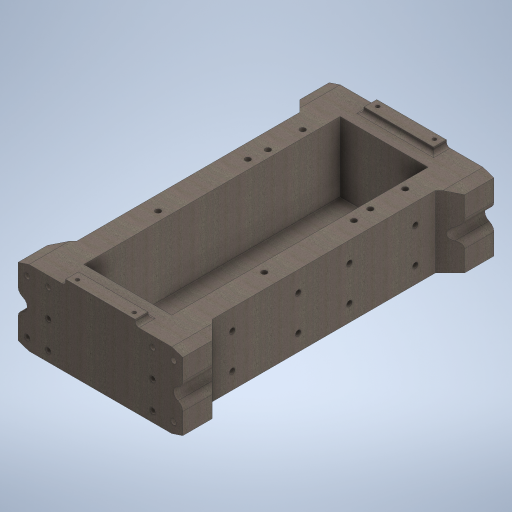
# Autodesk Inventor part: Part1
Saved by Autodesk Inventor 2023 (Build 270158000, 158)
## iProperties
Created: 2023-08-12
Part Number: Part1
Material: ABS Plastic
Document SubType Name: Modeling
Designer: Dawid
Density: 1.06 g/cm^3
Appearance: Walnut
Author: Dawid
Autodesk Inventor part; units mm, degrees
ref_plane "YZ Plane" through (0, 0, 0) normal (1, 0, 0) x (0, 1, 0)
ref_plane "XZ Plane" through (0, 0, 0) normal (0, 1, 0) x (-1, 0, 0)
ref_plane "XY Plane" through (0, 0, 0) normal (0, 0, 1) x (1, 0, 0)
sketch "Sketch1" plane through (0, 0, 0) normal (0, 1, 0) x (-1, 0, 0)
  line L0 (45, 85) -> (-45, 85)
  line L1 (-45, 85) -> (-45, -85)
  line L2 (-45, -85) -> (45, -85)
  line L3 (45, -85) -> (45, 85)
  line L4 (45, 85) -> (-45, -85) construction
  line L5 (-45, 85) -> (45, -85) construction
  line L6 (24, 70) -> (-24, 70)
  line L7 (-24, 70) -> (-24, -70)
  line L8 (-24, -70) -> (24, -70)
  line L9 (24, -70) -> (24, 70)
  line L10 (24, 70) -> (-24, -70) construction
  line L11 (-24, 70) -> (24, -70) construction
  point P0 (0, 0)
  dimension "d0" = 90
  dimension "d1" = 170
  dimension "d2" = 48
  dimension "d3" = 140
  constraints: 24 end point, 4 midpoint, 4 parallel, 2 horizontal, 2 perpendicular
  measures "d0" distance of L2.end L1.end
  measures "d1" distance of L1.end L0.end
  measures "d2" distance of L8.end L7.end
  measures "d3" distance of L7.end L6.end
extrude "Extrusion1" add sketch "Sketch1" along normal blind 38
sketch "Sketch2" plane through (0, 0, 0) normal (0, -1, 0) x (1, 0, 0)
  line L0 (45, 85) -> (45, -85) projected
  line L1 (-45, -85) -> (-45, 85) projected
  line L2 (45, 85) -> (-45, 85)
  line L3 (-45, 85) -> (-45, -85)
  line L4 (-45, -85) -> (45, -85)
  line L5 (45, -85) -> (45, 85)
  point P0 (0, 0)
  constraints: 8 end point, 2 parallel, 1 horizontal, 1 perpendicular
extrude "Extrusion2" add sketch "Sketch2" along normal blind 3
sketch "Sketch4" plane through (0, 38, 0) normal (0, 1, 0) x (1, 0, 0)
  line L0 (-29, -24.5) -> (29, -24.5)
  line L1 (29, -24.5) -> (29, 24.5)
  line L2 (29, 24.5) -> (-29, 24.5)
  line L3 (-29, 24.5) -> (-29, -24.5)
  line L4 (-29, -24.5) -> (29, 24.5) construction
  line L5 (29, -24.5) -> (-29, 24.5) construction
  circle A0 centre (-29, -24.5) radius 1.5
  circle A1 centre (-29, 24.5) radius 1.5
  circle A2 centre (29, 24.5) radius 1.5
  circle A3 centre (29, -24.5) radius 1.5
  point P0 (0, 0)
  dimension "d8" = 58
  dimension "d9" = 49
  dimension "d10" = 3
  dimension "d11" = 3
  dimension "d12" = 3
  dimension "d13" = 3
  constraints: 12 end point, 4 centre point, 4 coincident, 2 midpoint, 2 parallel, 1 horizontal, 1 perpendicular
  measures "d8" distance of L2.end L1.end
  measures "d9" distance of L1.end L0.end
  measures "d10" diameter of A0
  measures "d11" diameter of A1
  measures "d12" diameter of A2
  measures "d13" diameter of A3
extrude "Extrusion3" cut sketch "Sketch4" against normal blind 7 contours L3 A0 L0 | L0 A0 L3 | A3 L1 L0 | L0 L1 A3 | A1 L2 L3 | L3 L2 A1 | A2 L2 L1 | L1 L2 A2
sketch "Sketch5" plane through (0, 38, 0) normal (0, 1, 0) x (1, 0, 0)
  line L0 (0, 0) -> (0, 24.5)
  line L1 (0, 24.5) -> (0, 34.5)
  line L2 (0, 34.5) -> (-28, 34.5)
  line L3 (-28, 34.5) -> (28, 34.5)
  line L4 (28, 34.5) -> (28, 53.5)
  line L5 (28, 53.5) -> (-28, 53.5)
  line L6 (-28, 53.5) -> (-28, 34.5)
  circle A0 centre (-28, 34.5) radius 1.5
  circle A1 centre (-28, 53.5) radius 1.5
  circle A2 centre (28, 53.5) radius 1.5
  circle A3 centre (28, 34.5) radius 1.5
  dimension "d16" = 10
  dimension "d17" = 28
  dimension "d18" = 56
  dimension "d19" = 19
  dimension "d20" = 3
  dimension "d21" = 3
  dimension "d22" = 3
  dimension "d23" = 3
  constraints: 14 end point, 4 centre point, 4 coincident, 4 perpendicular, 2 point on line, 1 vertical
  measures "d16" distance of L0.end L1.end
  measures "d17" distance of L1.end L2.end
  measures "d18" distance of L2.end L3.end
  measures "d19" distance of L3.end L4.end
  measures "d20" diameter of A0
  measures "d21" diameter of A1
  measures "d22" diameter of A2
  measures "d23" diameter of A3
extrude "Extrusion4" cut sketch "Sketch5" against normal blind 7 contours A0 L6 L2 | L2 L6 A0 | A3 L4 L3 | L3 L4 A3 | A1 L5 L6 | L6 L5 A1 | A2 L5 L4 | L4 L5 A2
sketch "Sketch7" plane through (45, 38, -85) normal (0, 0, -1) x (-1, 0, 0)
  line L0 (90, -41) -> (90, 0) projected
  line L1 (90, -41) -> (0, -41) projected
  line L2 (21.5, 0) -> (68.5, 0)
  line L3 (68.5, 0) -> (68.5, -41)
  line L4 (68.5, -41) -> (21.5, -41)
  line L5 (21.5, -41) -> (21.5, 0)
  line L6 (21.5, 0) -> (68.5, -41) construction
  line L7 (68.5, 0) -> (21.5, -41) construction
  line L8 (0, 0) -> (90, 0)
  line L9 (90, 0) -> (90, -41)
  line L10 (90, -41) -> (0, -41)
  line L11 (0, -41) -> (0, 0)
  line L12 (0, 0) -> (90, -41) construction
  line L13 (90, 0) -> (0, -41) construction
  line L14 (11.5, 0) -> (78.5, 0)
  line L15 (78.5, 0) -> (78.5, -41)
  line L16 (78.5, -41) -> (11.5, -41)
  line L17 (11.5, -41) -> (11.5, 0)
  line L18 (11.5, 0) -> (78.5, -41) construction
  line L19 (78.5, 0) -> (11.5, -41) construction
  line L20 (0, 0) -> (0, -20.5)
  line L21 (0, -41) -> (0, 0) projected
  line L22 (0, -20.5) -> (90, -20.5)
  line L23 (-8.5, 0) -> (98.5, 0)
  line L24 (98.5, 0) -> (98.5, -41)
  line L25 (98.5, -41) -> (-8.5, -41)
  line L26 (-8.5, -41) -> (-8.5, 0)
  line L27 (-8.5, 0) -> (98.5, -41) construction
  line L28 (98.5, 0) -> (-8.5, -41) construction
  line L29 (-8.5, 0) -> (1.5, 0)
  line L30 (0, 0) -> (90, 0) projected
  line L31 (1.5, 0) -> (1.5, -41)
  line L32 (98.5, -41) -> (88.5, -41)
  line L33 (88.5, -41) -> (88.5, 0)
  circle A0 centre (1.5, -20.5) radius 10
  circle A1 centre (88.5, -20.5) radius 10
  line L34 (21.5, -41) -> (16.5, -41)
  line L35 (16.5, -41) -> (16.5, 0)
  line L36 (16.5, -20.5) -> (16.5, -35.5)
  line L37 (16.5, -35.5) -> (16.5, -5.5)
  circle A2 centre (16.5, -5.5) radius 1.5
  circle A3 centre (16.5, -35.5) radius 1.5
  circle A4 centre (16.5, -20.5) radius 1.5
  line L38 (0, 0) -> (5, 0)
  line L39 (5, 0) -> (5, -6)
  line L40 (0, -41) -> (5, -41)
  line L41 (5, -41) -> (5, -35)
  circle A5 centre (5, -35) radius 1.5
  circle A6 centre (5, -6) radius 1.5
  line L42 (68.5, -20.5) -> (73.5, -20.5)
  line L43 (73.5, -20.5) -> (73.5, -35.5)
  line L44 (73.5, -35.5) -> (73.5, -5.5)
  line L45 (90, 0) -> (85, 0)
  line L46 (85, 0) -> (85, -6)
  line L47 (90, -41) -> (85, -41)
  line L48 (85, -41) -> (85, -35)
  circle A7 centre (73.5, -5.5) radius 1.5
  circle A8 centre (73.5, -20.5) radius 1.5
  circle A9 centre (73.5, -35.5) radius 1.5
  circle A10 centre (85, -35) radius 1.5
  circle A11 centre (85, -6) radius 1.5
  point P0 (45, -38)
  point P1 (45, -20.5)
  point P2 (45, -20.5)
  dimension "d27" = 47
  dimension "d28" = 67
  dimension "d29" = 107
  dimension "d30" = 10
  dimension "d31" = 10
  dimension "d32" = 5
  dimension "d33" = 15
  dimension "d34" = 30
  dimension "d35" = 3
  dimension "d36" = 3
  dimension "d37" = 3
  dimension "d38" = 5
  dimension "d39" = 6
  dimension "d40" = 5
  dimension "d41" = 6
  dimension "d42" = 3
  dimension "d43" = 3
  dimension "d44" = 5
  dimension "d45" = 15
  dimension "d46" = 30
  dimension "d47" = 5
  dimension "d48" = 6
  dimension "d49" = 5
  dimension "d50" = 6
  dimension "d51" = 3
  dimension "d52" = 3
  dimension "d53" = 3
  dimension "d54" = 3
  dimension "d55" = 3
  constraints: 90 end point, 14 midpoint, 13 point on line, 12 centre point, 11 perpendicular, 10 coincident, 8 parallel, 4 horizontal, 1 tangent, 1 vertical, 5 other
  measures "d27" distance of L3.end L4.end
  measures "d28" distance of L15.end L16.end
  measures "d29" distance of L24.end L25.end
  measures "d30" distance of L23.start L29.end
  measures "d31" distance of L24.end L32.end
  measures "d32" distance of L4.end L34.end
  measures "d33" distance of L36.start L36.end
  measures "d34" distance of L36.end L37.end
  measures "d35" diameter of A2
  measures "d36" diameter of A3
  measures "d37" diameter of A4
  measures "d38" distance of L20.start L38.end
  measures "d39" distance of L38.end L39.end
  measures "d40" distance of L10.end L40.end
  measures "d41" distance of L40.end L41.end
  measures "d42" diameter of A5
  measures "d43" diameter of A6
  measures "d44" distance of L42.start L42.end
  measures "d45" distance of L42.end L43.end
  measures "d46" distance of L43.end L44.end
  measures "d47" distance of L8.end L45.end
  measures "d48" distance of L45.end L46.end
  measures "d49" distance of L0.start L47.end
  measures "d50" distance of L47.end L48.end
  measures "d51" diameter of A7
  measures "d52" diameter of A8
  measures "d53" diameter of A9
  measures "d54" diameter of A10
  measures "d55" diameter of A11
extrude "Extrusion5" cut sketch "Sketch7" against normal blind 8 contours A8 L43 L22 | L22 L44 A8 | L43 A8 L22 | L22 A8 L44 | A3 L35 | L35 A3 | A4 L35 L22 | L22 L35 A4 | A2 L35 | L35 A2 | L35 A4 L22 | L22 A4 L35 | A5 | A6 | A7 | A9 | A10 | A11
sketch "Sketch8" plane through (-45, 38, 85) normal (0, 0, 1) x (1, 0, 0)
  line L0 (90, -41) -> (90, 0)
  line L1 (90, -41) -> (0, -41)
  line L2 (21.5, 0) -> (68.5, 0)
  line L3 (68.5, 0) -> (68.5, -41)
  line L4 (68.5, -41) -> (21.5, -41)
  line L5 (21.5, -41) -> (21.5, 0)
  line L6 (21.5, 0) -> (68.5, -41) construction
  line L7 (68.5, 0) -> (21.5, -41) construction
  line L8 (0, 0) -> (90, 0)
  line L9 (90, 0) -> (90, -41)
  line L10 (90, -41) -> (0, -41)
  line L11 (0, -41) -> (0, 0)
  line L12 (0, 0) -> (90, -41) construction
  line L13 (90, 0) -> (0, -41) construction
  line L14 (11.5, 0) -> (78.5, 0)
  line L15 (78.5, 0) -> (78.5, -41)
  line L16 (78.5, -41) -> (11.5, -41)
  line L17 (11.5, -41) -> (11.5, 0)
  line L18 (11.5, 0) -> (78.5, -41) construction
  line L19 (78.5, 0) -> (11.5, -41) construction
  line L20 (0, 0) -> (0, -20.5)
  line L21 (0, -41) -> (0, 0)
  line L22 (0, -20.5) -> (90, -20.5)
  line L23 (-8.5, 0) -> (98.5, 0)
  line L24 (98.5, 0) -> (98.5, -41)
  line L25 (98.5, -41) -> (-8.5, -41)
  line L26 (-8.5, -41) -> (-8.5, 0)
  line L27 (-8.5, 0) -> (98.5, -41) construction
  line L28 (98.5, 0) -> (-8.5, -41) construction
  line L29 (-8.5, 0) -> (1.5, 0)
  line L30 (0, 0) -> (90, 0)
  line L31 (1.5, 0) -> (1.5, -41)
  line L32 (98.5, -41) -> (88.5, -41)
  line L33 (88.5, -41) -> (88.5, 0)
  circle A0 centre (1.5, -20.5) radius 10
  circle A1 centre (88.5, -20.5) radius 10
  line L34 (21.5, -41) -> (16.5, -41)
  line L35 (16.5, -41) -> (16.5, 0)
  line L36 (16.5, -20.5) -> (16.5, -35.5)
  line L37 (16.5, -35.5) -> (16.5, -5.5)
  circle A2 centre (16.5, -5.5) radius 1.5
  circle A3 centre (16.5, -35.5) radius 1.5
  circle A4 centre (16.5, -20.5) radius 1.5
  line L38 (0, 0) -> (5, 0)
  line L39 (5, 0) -> (5, -6)
  line L40 (0, -41) -> (5, -41)
  line L41 (5, -41) -> (5, -35)
  circle A5 centre (5, -35) radius 1.5
  circle A6 centre (5, -6) radius 1.5
  line L42 (68.5, -20.5) -> (73.5, -20.5)
  line L43 (73.5, -20.5) -> (73.5, -35.5)
  line L44 (73.5, -35.5) -> (73.5, -5.5)
  line L45 (90, 0) -> (85, 0)
  line L46 (85, 0) -> (85, -6)
  line L47 (90, -41) -> (85, -41)
  line L48 (85, -41) -> (85, -35)
  circle A7 centre (73.5, -5.5) radius 1.5
  circle A8 centre (73.5, -20.5) radius 1.5
  circle A9 centre (73.5, -35.5) radius 1.5
  circle A10 centre (85, -35) radius 1.5
  circle A11 centre (85, -6) radius 1.5
  point P0 (45, -38)
  point P1 (45, -38)
  point P2 (45, -20.5)
  point P3 (45, -20.5)
  dimension "d58" = 47
  dimension "d59" = 67
  dimension "d60" = 107
  dimension "d61" = 10
  dimension "d62" = 10
  dimension "d63" = 5
  dimension "d64" = 15
  dimension "d65" = 30
  dimension "d66" = 3
  dimension "d67" = 3
  dimension "d68" = 3
  dimension "d69" = 5
  dimension "d70" = 6
  dimension "d71" = 5
  dimension "d72" = 6
  dimension "d73" = 3
  dimension "d74" = 3
  dimension "d75" = 5
  dimension "d76" = 15
  dimension "d77" = 30
  dimension "d78" = 5
  dimension "d79" = 6
  dimension "d80" = 5
  dimension "d81" = 6
  dimension "d82" = 3
  dimension "d83" = 3
  dimension "d84" = 3
  dimension "d85" = 3
  dimension "d86" = 3
  constraints: 96 end point, 14 midpoint, 13 point on line, 12 centre point, 11 perpendicular, 10 coincident, 8 parallel, 4 horizontal, 1 tangent, 1 vertical, 7 other
  measures "d58" distance of L6.end L7.end
  measures "d59" distance of L15.end L19.end
  measures "d60" distance of L24.end L28.end
  measures "d61" distance of L27.start L31.start
  measures "d62" distance of L24.end L33.start
  measures "d63" distance of L7.end L35.start
  measures "d64" distance of L36.start L37.start
  measures "d65" distance of L37.start L37.end
  measures "d66" diameter of A2
  measures "d67" diameter of A3
  measures "d68" diameter of A4
  measures "d69" distance of L20.start L39.start
  measures "d70" distance of L39.start L39.end
  measures "d71" distance of L10.end L40.end
  measures "d72" distance of L40.end L41.end
  measures "d73" diameter of A5
  measures "d74" diameter of A6
  measures "d75" distance of L42.start L42.end
  measures "d76" distance of L42.end L44.start
  measures "d77" distance of L44.start L44.end
  measures "d78" distance of L9.start L46.start
  measures "d79" distance of L46.start L46.end
  measures "d80" distance of L0.start L48.start
  measures "d81" distance of L48.start L48.end
  measures "d82" diameter of A7
  measures "d83" diameter of A8
  measures "d84" diameter of A9
  measures "d85" diameter of A10
  measures "d86" diameter of A11
extrude "Extrusion6" cut sketch "Sketch8" against normal blind 8 contours A8 L43 L22 | L22 L44 A8 | L43 A8 L22 | L22 A8 L44 | A3 L35 | L35 A3 | A4 L35 L22 | L22 L35 A4 | A2 L35 | L35 A2 | L35 A4 L22 | L22 A4 L35 | A5 | A6 | A7 | A9 | A10 | A11
sketch "Sketch10" plane through (-45, 38, -85) normal (-1, 0, 0) x (0, 0, 1)
  line L0 (0, -41) -> (0, 0) projected
  line L1 (0, 0) -> (85, 0)
  line L2 (15, 0) -> (155, 0) projected
  line L3 (0, -41) -> (170, -41) projected
  line L4 (15, -38) -> (15, 0) projected
  line L5 (25, 0) -> (145, 0)
  line L6 (145, -41) -> (25, -41)
  line L7 (20, 0) -> (150, 0)
  line L8 (150, 0) -> (150, -41)
  line L9 (150, -41) -> (20, -41)
  line L10 (20, -41) -> (20, 0)
  point P0 (85, -38)
  dimension "d91" = 130
  constraints: 14 end point, 3 parallel, 2 horizontal, 2 point on line, 1 midpoint, 1 perpendicular
  measures "d91" distance of L8.end L9.end
extrude "Extrusion7" cut sketch "Sketch10" against normal blind 8 contours L10 L1 L2 L8 L3
chamfer "Chamfer1" distance 4 angle 45 4 edges at (-37, 17.5, -65) (-37, 17.5, 65) (-45, 17.5, 65) (-45, 17.5, -65)
sketch "Sketch11" plane through (45, 38, 85) normal (1, 0, 0) x (0, 0, -1)
  line L0 (170, -41) -> (0, -41) projected
  line L1 (170, -41) -> (170, 0) projected
  line L2 (170, -41) -> (170, 0)
  line L3 (170, 0) -> (170, -20.5)
  line L4 (170, -20.5) -> (0, -20.5)
  line L5 (0, -41) -> (0, 0) projected
  line L6 (0, 0) -> (170, 0) projected
  line L7 (150, -41) -> (20, -41)
  line L8 (20, -41) -> (20, 0)
  line L9 (20, 0) -> (150, 0)
  line L10 (150, 0) -> (150, -41)
  line L11 (150, -41) -> (20, 0) construction
  line L12 (20, -41) -> (150, 0) construction
  point P0 (85, -38)
  point P1 (85, -20.5)
  dimension "d97" = 130
  constraints: 18 end point, 5 midpoint, 3 equal length, 1 horizontal, 1 perpendicular, 1 point on line
  measures "d97" distance of L8.end L9.end
extrude "Extrusion8" cut sketch "Sketch11" against normal blind 8 contours L0 L8 L4 L10 | L4 L8 L6 L10
chamfer "Chamfer2" distance 4 angle 45 4 edges at (37, 17.5, -65) (45, 17.5, -65) (45, 17.5, 65) (37, 17.5, 65)
sketch "Sketch13" plane through (37, 38, 85) normal (1, 0, 0) x (0, 0, -1)
  line L0 (0, 0) -> (16, 0) projected
  line L1 (0, 0) -> (0, -20.5)
  line L2 (0, -41) -> (0, 0) projected
  line L3 (0, -20.5) -> (170, -20.5)
  line L4 (85, -20.5) -> (85, -41)
  line L5 (24, -41) -> (146, -41) projected
  line L6 (85, -20.5) -> (90, -20.5)
  line L7 (90, -20.5) -> (80, -20.5)
  line L8 (26, -8.5) -> (144, -8.5)
  line L9 (144, -8.5) -> (144, -32.5)
  line L10 (144, -32.5) -> (26, -32.5)
  line L11 (26, -32.5) -> (26, -8.5)
  line L12 (26, -8.5) -> (144, -32.5) construction
  line L13 (144, -8.5) -> (26, -32.5) construction
  line L14 (80, -8.5) -> (90, -8.5)
  line L15 (90, -8.5) -> (90, -32.5)
  line L16 (90, -32.5) -> (80, -32.5)
  line L17 (80, -32.5) -> (80, -8.5)
  line L18 (80, -8.5) -> (90, -32.5) construction
  line L19 (90, -8.5) -> (80, -32.5) construction
  line L20 (80, -32.5) -> (80, -30)
  line L21 (80, -30) -> (71, -30)
  line L22 (80, -8.5) -> (80, -11)
  line L23 (80, -11) -> (71, -11)
  line L24 (26, -8.5) -> (26, -11)
  line L25 (26, -11) -> (35, -11)
  line L26 (26, -32.5) -> (26, -30)
  line L27 (26, -30) -> (35, -30)
  line L28 (90, -8.5) -> (90, -11)
  line L29 (90, -11) -> (99, -11)
  line L30 (90, -32.5) -> (90, -30)
  line L31 (90, -30) -> (99, -30)
  line L32 (144, -32.5) -> (144, -30)
  line L33 (144, -30) -> (135, -30)
  line L34 (144, -8.5) -> (144, -11)
  line L35 (144, -11) -> (135, -11)
  circle A0 centre (35, -11) radius 1.5
  circle A1 centre (35, -30) radius 1.5
  circle A2 centre (71, -30) radius 1.5
  circle A3 centre (71, -11) radius 1.5
  circle A4 centre (99, -11) radius 1.5
  circle A5 centre (135, -11) radius 1.5
  circle A6 centre (99, -30) radius 1.5
  circle A7 centre (135, -30) radius 1.5
  point P0 (85, -38)
  dimension "d103" = 5
  dimension "d104" = 10
  dimension "d105" = 118
  dimension "d106" = 24
  dimension "d107" = 2.5
  dimension "d108" = 9
  dimension "d109" = 2.5
  dimension "d110" = 9
  dimension "d111" = 2.5
  dimension "d112" = 9
  dimension "d113" = 2.5
  dimension "d114" = 9
  dimension "d115" = 2.5
  dimension "d116" = 9
  dimension "d117" = 2.5
  dimension "d118" = 9
  dimension "d119" = 2.5
  dimension "d120" = 9
  dimension "d121" = 2.5
  dimension "d122" = 9
  dimension "d123" = 3
  dimension "d124" = 3
  dimension "d125" = 3
  dimension "d126" = 3
  dimension "d127" = 3
  dimension "d128" = 3
  dimension "d129" = 3
  dimension "d130" = 3
  constraints: 66 end point, 11 point on line, 9 perpendicular, 8 centre point, 8 coincident, 7 midpoint, 5 parallel, 3 horizontal
  measures "d103" distance of L4.start L6.end
  measures "d104" distance of L6.end L7.end
  measures "d105" distance of L9.end L10.end
  measures "d106" distance of L8.end L9.end
  measures "d107" distance of L16.end L20.end
  measures "d108" distance of L20.end L21.end
  measures "d109" distance of L14.start L22.end
  measures "d110" distance of L22.end L23.end
  measures "d111" distance of L8.start L24.end
  measures "d112" distance of L24.end L25.end
  measures "d113" distance of L10.end L26.end
  measures "d114" distance of L26.end L27.end
  measures "d115" distance of L14.end L28.end
  measures "d116" distance of L28.end L29.end
  measures "d117" distance of L15.end L30.end
  measures "d118" distance of L30.end L31.end
  measures "d119" distance of L9.end L32.end
  measures "d120" distance of L32.end L33.end
  measures "d121" distance of L8.end L34.end
  measures "d122" distance of L34.end L35.end
  measures "d123" diameter of A0
  measures "d124" diameter of A1
  measures "d125" diameter of A2
  measures "d126" diameter of A3
  measures "d127" diameter of A4
  measures "d128" diameter of A5
  measures "d129" diameter of A6
  measures "d130" diameter of A7
extrude "Extrusion9" cut sketch "Sketch13" against normal blind 5 contours A0 | A1 | A2 | A3 | A4 | A5 | A6 | A7
sketch "Sketch14" plane through (-37, 38, -85) normal (-1, 0, 0) x (0, 0, 1)
  line L0 (0, 0) -> (16, 0)
  line L1 (0, 0) -> (0, -20.5)
  line L2 (0, -41) -> (0, 0)
  line L3 (0, -20.5) -> (170, -20.5)
  line L4 (85, -20.5) -> (85, -41)
  line L5 (24, -41) -> (146, -41)
  line L6 (85, -20.5) -> (90, -20.5)
  line L7 (90, -20.5) -> (80, -20.5)
  line L8 (26, -8.5) -> (144, -8.5)
  line L9 (144, -8.5) -> (144, -32.5)
  line L10 (144, -32.5) -> (26, -32.5)
  line L11 (26, -32.5) -> (26, -8.5)
  line L12 (26, -8.5) -> (144, -32.5) construction
  line L13 (144, -8.5) -> (26, -32.5) construction
  line L14 (80, -8.5) -> (90, -8.5)
  line L15 (90, -8.5) -> (90, -32.5)
  line L16 (90, -32.5) -> (80, -32.5)
  line L17 (80, -32.5) -> (80, -8.5)
  line L18 (80, -8.5) -> (90, -32.5) construction
  line L19 (90, -8.5) -> (80, -32.5) construction
  line L20 (80, -32.5) -> (80, -30)
  line L21 (80, -30) -> (71, -30)
  line L22 (80, -8.5) -> (80, -11)
  line L23 (80, -11) -> (71, -11)
  line L24 (26, -8.5) -> (26, -11)
  line L25 (26, -11) -> (35, -11)
  line L26 (26, -32.5) -> (26, -30)
  line L27 (26, -30) -> (35, -30)
  line L28 (90, -8.5) -> (90, -11)
  line L29 (90, -11) -> (99, -11)
  line L30 (90, -32.5) -> (90, -30)
  line L31 (90, -30) -> (99, -30)
  line L32 (144, -32.5) -> (144, -30)
  line L33 (144, -30) -> (135, -30)
  line L34 (144, -8.5) -> (144, -11)
  line L35 (144, -11) -> (135, -11)
  circle A0 centre (35, -11) radius 1.5
  circle A1 centre (35, -30) radius 1.5
  circle A2 centre (71, -30) radius 1.5
  circle A3 centre (71, -11) radius 1.5
  circle A4 centre (99, -11) radius 1.5
  circle A5 centre (135, -11) radius 1.5
  circle A6 centre (99, -30) radius 1.5
  circle A7 centre (135, -30) radius 1.5
  point P0 (85, -38)
  point P1 (85, -38)
  dimension "d133" = 5
  dimension "d134" = 10
  dimension "d135" = 118
  dimension "d136" = 24
  dimension "d137" = 2.5
  dimension "d138" = 9
  dimension "d139" = 2.5
  dimension "d140" = 9
  dimension "d141" = 2.5
  dimension "d142" = 9
  dimension "d143" = 2.5
  dimension "d144" = 9
  dimension "d145" = 2.5
  dimension "d146" = 9
  dimension "d147" = 2.5
  dimension "d148" = 9
  dimension "d149" = 2.5
  dimension "d150" = 9
  dimension "d151" = 2.5
  dimension "d152" = 9
  dimension "d153" = 3
  dimension "d154" = 3
  dimension "d155" = 3
  dimension "d156" = 3
  dimension "d157" = 3
  dimension "d158" = 3
  dimension "d159" = 3
  dimension "d160" = 3
  constraints: 72 end point, 11 point on line, 9 perpendicular, 8 centre point, 8 coincident, 7 midpoint, 5 parallel, 3 horizontal
  measures "d133" distance of L4.start L7.start
  measures "d134" distance of L7.start L7.end
  measures "d135" distance of L12.end L10.end
  measures "d136" distance of L8.end L12.end
  measures "d137" distance of L17.start L20.end
  measures "d138" distance of L20.end L21.end
  measures "d139" distance of L14.start L22.end
  measures "d140" distance of L22.end L23.end
  measures "d141" distance of L8.start L25.start
  measures "d142" distance of L25.start L25.end
  measures "d143" distance of L10.end L26.end
  measures "d144" distance of L26.end L27.end
  measures "d145" distance of L14.end L28.end
  measures "d146" distance of L28.end L29.end
  measures "d147" distance of L18.end L31.start
  measures "d148" distance of L31.start L31.end
  measures "d149" distance of L12.end L32.end
  measures "d150" distance of L32.end L33.end
  measures "d151" distance of L8.end L34.end
  measures "d152" distance of L34.end L35.end
  measures "d153" diameter of A0
  measures "d154" diameter of A1
  measures "d155" diameter of A2
  measures "d156" diameter of A3
  measures "d157" diameter of A4
  measures "d158" diameter of A5
  measures "d159" diameter of A6
  measures "d160" diameter of A7
extrude "Extrusion10" cut sketch "Sketch14" against normal blind 5 contours A0 | A1 | A2 | A3 | A4 | A5 | A6 | A7
sketch "Sketch15" plane through (0, 38, 0) normal (0, 1, 0) x (1, 0, 0)
  line L0 (45, -85) -> (-45, -85) projected
  line L1 (-45, -85) -> (45, -85)
  line L2 (0, -85) -> (0, -78)
  line L3 (0, -78) -> (-19, -78)
  line L4 (-19, -78) -> (19, -78)
  line L5 (19, -78) -> (19, -85)
  line L6 (-19, -78) -> (-19, -85)
  point P0 (0, 0)
  dimension "d163" = 7
  dimension "d164" = 19
  dimension "d165" = 38
  constraints: 12 end point, 3 perpendicular, 3 point on line, 1 collinear, 1 midpoint, 1 vertical
  measures "d163" distance of L2.start L2.end
  measures "d164" distance of L2.end L3.end
  measures "d165" distance of L3.end L4.end
extrude "Extrusion11" add sketch "Sketch15" along normal blind 3
sketch "Sketch16" plane through (0, 38, 0) normal (0, 1, 0) x (1, 0, 0)
  line L0 (45, -85) -> (-45, -85)
  line L1 (-45, -85) -> (45, -85)
  line L2 (0, -85) -> (0, -78)
  line L3 (0, -78) -> (-19, -78)
  line L4 (-19, -78) -> (19, -78)
  line L5 (19, -78) -> (19, -85)
  line L6 (-19, -78) -> (-19, -85)
  line L7 (45, 85) -> (-45, 85) projected
  line L8 (0, 85) -> (0, 78)
  line L9 (0, 78) -> (19, 78)
  line L10 (19, 78) -> (-19, 78)
  line L11 (-19, 78) -> (-19, 85)
  line L12 (19, 78) -> (19, 85)
  point P0 (0, 0)
  dimension "d168" = 7
  dimension "d169" = 19
  dimension "d170" = 38
  dimension "d171" = 7
  dimension "d172" = 19
  dimension "d173" = 38
  constraints: 24 end point, 6 point on line, 5 perpendicular, 2 equal length, 2 midpoint, 2 vertical
  measures "d168" distance of L2.start L2.end
  measures "d169" distance of L2.end L3.end
  measures "d170" distance of L3.end L4.end
  measures "d171" distance of L8.start L8.end
  measures "d172" distance of L8.end L9.end
  measures "d173" distance of L9.end L10.end
extrude "Extrusion12" add sketch "Sketch16" along normal blind 3 contours L12 L9 L8 L7 | L8 L10 L11 L7
sketch "Sketch17" plane through (0, 41, 0) normal (0, 1, 0) x (1, 0, 0)
  line L0 (45, -85) -> (-45, -85) projected
  line L1 (0, -85) -> (0, -82)
  line L2 (0, -82) -> (-15.5, -82)
  line L3 (-15.5, -82) -> (15.5, -82)
  circle A0 centre (-15.5, -82) radius 1
  circle A1 centre (15.5, -82) radius 1
  line L4 (-45, 85) -> (45, 85) projected
  line L5 (0, 85) -> (0, 82)
  line L6 (0, 82) -> (-15.5, 82)
  line L7 (-15.5, 82) -> (15.5, 82)
  circle A2 centre (-15.5, 82) radius 1
  circle A3 centre (15.5, 82) radius 1
  point P0 (0, 0)
  dimension "d176" = 3
  dimension "d177" = 15.5
  dimension "d178" = 31
  dimension "d179" = 2
  dimension "d180" = 2
  dimension "d181" = 3
  dimension "d182" = 15.5
  dimension "d183" = 31
  dimension "d184" = 2
  dimension "d185" = 2
  constraints: 12 end point, 4 centre point, 4 coincident, 2 midpoint, 2 perpendicular, 2 point on line, 2 vertical
  measures "d176" distance of L1.start L1.end
  measures "d177" distance of L1.end L2.end
  measures "d178" distance of L2.end L3.end
  measures "d179" diameter of A0
  measures "d180" diameter of A1
  measures "d181" distance of L5.start L5.end
  measures "d182" distance of L5.end L6.end
  measures "d183" distance of L6.end L7.end
  measures "d184" diameter of A2
  measures "d185" diameter of A3
extrude "Extrusion13" cut sketch "Sketch17" against normal blind 6
chamfer "Chamfer3" distance 6 distance2 2 18 edges at (37, -3, 0) (43.0001, -3, 66.9999) (41, -3, 65) (39, -3, 63.0001) (39, -3, -63.0001) (41, -3, -65) (43.0001, -3, -66.9999) (45, -3, -76.9999) (45, -3, 77) (-37, -3, 0) (-39, -3, -63.0001) (-41, -3, -65) (-43.0001, -3, -66.9999) (-45, -3, -77) (-45, -3, 76.9999) (-43.0001, -3, 66.9999) (-41, -3, 65) (-39, -3, 63.0001) measured on face at (38.6464, -3, 63.3536) measured on face at (-38.6464, -3, 63.3536) measured on face at (-41, -3, -65.5) measured on face at (36.5, -3, 0) measured on face at (-42.6465, -3, -67.3535) measured on face at (42.6465, -3, -67.3535) measured on face at (-36.5, -3, 0) measured on face at (41, -3, -65.5) measured on face at (-44.5, -3, -77) measured on face at (42.6465, -3, 67.3535) measured on face at (-42.6465, -3, 67.3535) measured on face at (-44.5, -3, 77) measured on face at (44.5, -3, -77) measured on face at (-38.6464, -3, -63.3536) measured on face at (44.5, -3, 77) measured on face at (-41, -3, 65.5) measured on face at (38.6464, -3, -63.3536) measured on face at (41, -3, 65.5)
sketch "Sketch20" plane through (-19, 41, 85) normal (0, 0, 1) x (1, 0, 0)
  circle A0 centre (-9.5, -23.5) radius 1.5 projected
  line L0 (-9.5, -23.5) -> (-24.5, -23.5)
  circle A1 centre (-24.5, -23.5) radius 10
  circle A2 centre (47.5, -23.5) radius 1.5 projected
  line L1 (47.5, -23.5) -> (62.5, -23.5)
  circle A3 centre (62.5, -23.5) radius 10
  circle A4 centre (-24.5, -23.5) radius 3.5
  circle A5 centre (62.5, -23.5) radius 3.5
  point P0 (19, -41)
  dimension "d191" = 15
  dimension "d192" = 20
  dimension "d193" = 15
  dimension "d194" = 20
  dimension "d195" = 7
  dimension "d196" = 7
  constraints: 4 centre point, 4 coincident, 4 end point, 2 horizontal
  measures "d191" distance of L0.start L0.end
  measures "d192" diameter of A1
  measures "d193" distance of L1.start L1.end
  measures "d194" diameter of A3
  measures "d195" diameter of A4
  measures "d196" diameter of A5
extrude "Extrusion14" cut sketch "Sketch20" against normal blind 200 contours A4 | A5
fillet "Fillet1" radius 4 8 edges at (45, 20.6623, 76.9999) (45, 14.3377, 76.9999) (45, 14.3377, -77) (45, 20.6623, -77) (-45, 20.6623, 76.9999) (-45, 14.3377, 76.9999) (-45, 20.6623, -77) (-45, 14.3377, -77)
chamfer "Chamfer4" distance 6 distance2 2 4 edges at (45, 38, 76.9999) (45, 38, -77) (-45, 38, -76.9999) (-45, 38, 77) measured on face at (44.5, 38, 77) measured on face at (-44.5, 38, 77) measured on face at (-44.5, 38, -77) measured on face at (44.5, 38, -77)
fillet "Fillet2" radius 2 3 edges at (-19, 38, 81.5) (0, 38, 78) (19, 38, 81.5)
fillet "Fillet3" radius 2 3 edges at (0, 38, -78) (-19, 38, -81.5) (19, 38, -81.5)
body "Solid1"
